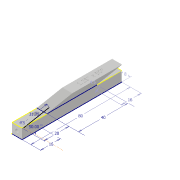
# Autodesk Inventor part: MineralStop1.25x50
Saved by Autodesk Inventor 2018 (Build 220112000, 112)
## iProperties
Created: 2018-12-12
Part Number: MineralStop1.25x50
Material: Generic
Document SubType Name: Modeling
Designer: ball
Density: 1 g/cm^3
Appearance: Default
Author: ball
Autodesk Inventor part; units mm, degrees
ref_plane "YZ Plane" through (0, 0, 0) normal (1, 0, 0) x (0, 1, 0)
ref_plane "XZ Plane" through (0, 0, 0) normal (0, 1, 0) x (-1, 0, 0)
ref_plane "XY Plane" through (0, 0, 0) normal (0, 0, 1) x (1, 0, 0)
sketch "Sketch1" plane through (0, 0, 0) normal (0, 1, 0) x (-1, 0, 0)
  line L0 (0, 0) -> (-8, 0)
  line L1 (-8, 0) -> (-8, -80)
  line L2 (-8, -80) -> (0, -80)
  line L3 (0, -80) -> (0, 0)
  circle A0 centre (-4, -16) radius 2.25
  circle A1 centre (-4, -64) radius 2.25
  circle A2 centre (-4, -16) radius 3.5 construction
  dimension "d0" = 8
  dimension "d1" = 80
  dimension "d6" = 4.5
  dimension "d7" = 4.5
  dimension "d26" = 16
  dimension "d27" = 16
  dimension "d43" = 7
  constraints: 8 end point, 3 centre point, 2 parallel, 1 coincident, 1 horizontal, 1 perpendicular
  measures "d0" distance of L2.end L1.end
  measures "d1" distance of L1.end L0.end
  measures "d6" diameter of A0
  measures "d7" diameter of A1
  measures "d26" distance from line of L0 A0.centre
  measures "d27" distance from line of L2 A1.centre
  measures "d43" diameter of A2
extrude "Extrusion1" [suppressed]
extrude "Extrusion2" add sketch "Sketch1" along normal blind 8
sketch "Sketch2" plane through (0, 0, 0) normal (0, 0, 1) x (1, 0, 0)
  circle A0 centre (4, 4) radius 1.35
  point P0 (0, 0)
  dimension "d10" = 2.7
  constraints: 1 centre point
  measures "d10" diameter of A0
hole "Hole1" at (4, 4, 0) direction (0, 0, -1) diameter 2.7 depth 10
sketch "Sketch3" plane through (8, 0, -80) normal (0, 0, -1) x (-1, 0, 0)
  circle A0 centre (4, 4) radius 1.35
  point P0 (8, 0)
  dimension "d18" = 2.7
  constraints: 1 centre point
  measures "d18" diameter of A0
hole "Hole2" at (4, 4, -80) direction (0, 0, 1) diameter 2.7 depth 10
sketch "Sketch5" plane through (0, 0, 0) normal (0, 0, 1) x (1, 0, 0)
  line L0 (9.3659, 8.9784) -> (29.7744, 33.3003)
  line L1 (9.3659, 8.9784) -> (41.1159, 8.9784) construction
  point P0 (0, 0)
  dimension "d33" = 31.75
  dimension "d34" = 50
  constraints: 4 end point, 1 equal length, 1 horizontal
  measures "d33" distance of L0.start L0.end
  measures "d34" angle of L1 L0
sketch "Sketch4" plane through (0, 8, 0) normal (0, 1, 0) x (1, 0, 0)
  line L0 (0, 80) -> (0, 0) projected
  line L1 (8, 0) -> (8, 80) projected
  line L2 (0, 60) -> (8, 60)
  line L3 (8, 60) -> (8, 20)
  line L4 (8, 20) -> (0, 20)
  line L5 (0, 20) -> (0, 60)
  line L6 (0, 0) -> (8, 0) projected
  line L7 (8, 80) -> (0, 80) projected
  dimension "d28" = 40
  dimension "d29" = 20
  constraints: 8 end point, 2 parallel, 2 point on line, 1 horizontal, 1 perpendicular
  measures "d28" distance of L2.end L3.end
  measures "d29" distance between parallel lines of L6 L4
sweep "Sweep1" add profiles "Sketch4" path "Sketch5" contours L2 L1 L4 L0
sweep "Sweep2" [suppressed]
sketch "Sketch6" plane through (20.4085, 32.3219, -60) normal (0, 1, 0) x (1, 0, 0)
  line L0 (2.4072, -31.6899) -> (2.4072, -9.1748) construction
  line L1 (2.4072, -9.1748) -> (5.6553, -9.1748) construction
  line L2 (5.6553, -9.1748) -> (5.6553, -31.6899) construction
  line L3 (5.6553, -31.6899) -> (2.4072, -31.6899) construction
  line L4 (5.591, -29.741) -> (5.591, -31.228)
  line L5 (5.591, -31.228) -> (5.2798, -31.228)
  line L6 (5.2798, -31.228) -> (5.2798, -30.6747)
  line L7 (5.2798, -30.6747) -> (3.2371, -30.6747)
  line L8 (3.2371, -30.6747) -> (3.2371, -31.228)
  line L9 (3.2371, -31.228) -> (2.958, -31.228)
  spline S0 degree 2 poles (2.958, -31.228) (2.958, -30.9143) (2.7802, -30.6179) (2.5332, -30.5981) knots 0 0 0 1 2 2 2
  line L10 (2.5332, -30.5981) -> (2.5332, -30.282)
  line L11 (2.5332, -30.282) -> (5.2798, -30.282)
  line L12 (5.2798, -30.282) -> (5.2798, -29.741)
  line L13 (5.2798, -29.741) -> (5.591, -29.741)
  line L14 (5.591, -28.5258) -> (5.591, -29.0149)
  line L15 (5.591, -29.0149) -> (5.0081, -29.0149)
  line L16 (5.0081, -29.0149) -> (5.0081, -28.5258)
  line L17 (5.0081, -28.5258) -> (5.591, -28.5258)
  line L18 (5.591, -26.0311) -> (5.591, -27.9108)
  line L19 (5.591, -27.9108) -> (5.1588, -27.9108)
  spline S1 degree 2 poles (5.1588, -27.9108) (4.9686, -27.7082) (4.6154, -27.3476) (4.4252, -27.1747) knots 0 0 0 1 2 2 2
  spline S2 degree 2 poles (4.4252, -27.1747) (4.0423, -26.8264) (3.5829, -26.572) (3.3384, -26.572) knots 0 0 0 1 2 2 2
  spline S3 degree 2 poles (3.3384, -26.572) (3.21, -26.572) (3.0173, -26.6511) (2.9555, -26.7227) knots 0 0 0 1 2 2 2
  spline S4 degree 2 poles (2.9555, -26.7227) (2.8938, -26.7943) (2.832, -26.982) (2.832, -27.0957) knots 0 0 0 1 2 2 2
  spline S5 degree 2 poles (2.832, -27.0957) (2.832, -27.2043) (2.8864, -27.4266) (2.9284, -27.5279) knots 0 0 0 1 2 2 2
  spline S6 degree 2 poles (2.9284, -27.5279) (2.963, -27.6144) (3.0618, -27.7749) (3.0963, -27.8243) knots 0 0 0 1 2 2 2
  line L20 (3.0963, -27.8243) -> (3.0963, -27.8465)
  line L21 (3.0963, -27.8465) -> (2.6616, -27.8465)
  spline S7 degree 2 poles (2.6616, -27.8465) (2.5999, -27.7206) (2.4788, -27.2686) (2.4788, -27.066) knots 0 0 0 1 2 2 2
  spline S8 degree 2 poles (2.4788, -27.066) (2.4788, -26.6387) (2.9308, -26.157) (3.3162, -26.157) knots 0 0 0 1 2 2 2
  spline S9 degree 2 poles (3.3162, -26.157) (3.4965, -26.157) (3.7978, -26.241) (3.9263, -26.3151) knots 0 0 0 1 2 2 2
  spline S10 degree 2 poles (3.9263, -26.3151) (4.0596, -26.3892) (4.3215, -26.6041) (4.4474, -26.7227) knots 0 0 0 1 2 2 2
  spline S11 degree 2 poles (4.4474, -26.7227) (4.6574, -26.9153) (5.1069, -27.3871) (5.2378, -27.5279) knots 0 0 0 1 2 2 2
  line L22 (5.2378, -27.5279) -> (5.2378, -26.0311)
  line L23 (5.2378, -26.0311) -> (5.591, -26.0311)
  spline S12 degree 2 poles (4.6228, -23.776) (4.8426, -23.776) (5.2181, -23.9167) (5.3564, -24.0452) knots 0 0 0 1 2 2 2
  spline S13 degree 2 poles (5.3564, -24.0452) (5.4947, -24.1736) (5.6553, -24.5565) (5.6553, -24.7936) knots 0 0 0 1 2 2 2
  spline S14 degree 2 poles (5.6553, -24.7936) (5.6553, -25.011) (5.5589, -25.4358) (5.4824, -25.5914) knots 0 0 0 1 2 2 2
  line L24 (5.4824, -25.5914) -> (5.0501, -25.5914)
  line L25 (5.0501, -25.5914) -> (5.0501, -25.5618)
  spline S15 degree 2 poles (5.0501, -25.5618) (5.0847, -25.5148) (5.1736, -25.3395) (5.2131, -25.2333) knots 0 0 0 1 2 2 2
  spline S16 degree 2 poles (5.2131, -25.2333) (5.2551, -25.1122) (5.3021, -24.9122) (5.3021, -24.7862) knots 0 0 0 1 2 2 2
  spline S17 degree 2 poles (5.3021, -24.7862) (5.3021, -24.6627) (5.2131, -24.4305) (5.1168, -24.3465) knots 0 0 0 1 2 2 2
  spline S18 degree 2 poles (5.1168, -24.3465) (5.0254, -24.27) (4.7834, -24.1909) (4.6203, -24.1909) knots 0 0 0 1 2 2 2
  spline S19 degree 2 poles (4.6203, -24.1909) (4.4573, -24.1909) (4.2498, -24.2798) (4.1807, -24.3638) knots 0 0 0 1 2 2 2
  spline S20 degree 2 poles (4.1807, -24.3638) (4.1041, -24.4503) (4.0399, -24.7071) (4.0399, -24.8628) knots 0 0 0 1 2 2 2
  spline S21 degree 2 poles (4.0399, -24.8628) (4.0399, -25.0307) (4.0917, -25.3642) (4.114, -25.4654) knots 0 0 0 1 2 2 2
  line L26 (4.114, -25.4654) -> (2.543, -25.4654)
  line L27 (2.543, -25.4654) -> (2.543, -23.7932)
  line L28 (2.543, -23.7932) -> (2.9012, -23.7932)
  line L29 (2.9012, -23.7932) -> (2.9012, -25.0727)
  line L30 (2.9012, -25.0727) -> (3.7138, -25.0727)
  spline S22 degree 2 poles (3.7138, -25.0727) (3.704, -24.9986) (3.6965, -24.8553) (3.6965, -24.7961) knots 0 0 0 1 2 2 2
  spline S23 degree 2 poles (3.6965, -24.7961) (3.6965, -24.5614) (3.7731, -24.2378) (3.8867, -24.0896) knots 0 0 0 1 2 2 2
  spline S24 degree 2 poles (3.8867, -24.0896) (4.0004, -23.939) (4.3462, -23.776) (4.6228, -23.776) knots 0 0 0 1 2 2 2
  line L31 (2.4072, -22.1087) -> (3.5928, -22.1976)
  line L32 (3.5928, -22.1976) -> (3.5928, -22.4668)
  line L33 (3.5928, -22.4668) -> (2.4072, -22.5558)
  line L34 (2.4072, -22.5558) -> (2.4072, -22.1087)
  line L35 (2.4072, -22.8793) -> (3.5928, -22.9683)
  line L36 (3.5928, -22.9683) -> (3.5928, -23.2375)
  line L37 (3.5928, -23.2375) -> (2.4072, -23.3264)
  line L38 (2.4072, -23.3264) -> (2.4072, -22.8793)
  line L39 (5.591, -18.5123) -> (5.591, -18.9841)
  line L40 (5.591, -18.9841) -> (4.7315, -19.5399)
  line L41 (4.7315, -19.5399) -> (5.591, -20.1104)
  line L42 (5.591, -20.1104) -> (5.591, -20.5476)
  line L43 (5.591, -20.5476) -> (4.4573, -19.7548)
  line L44 (4.4573, -19.7548) -> (3.3038, -20.5402)
  line L45 (3.3038, -20.5402) -> (3.3038, -20.0685)
  line L46 (3.3038, -20.0685) -> (4.156, -19.5152)
  line L47 (4.156, -19.5152) -> (3.3038, -18.9495)
  line L48 (3.3038, -18.9495) -> (3.3038, -18.5123)
  line L49 (3.3038, -18.5123) -> (4.4326, -19.3003)
  line L50 (4.4326, -19.3003) -> (5.591, -18.5123)
  spline S25 degree 2 poles (4.6228, -15.1136) (4.8426, -15.1136) (5.2181, -15.2544) (5.3564, -15.3828) knots 0 0 0 1 2 2 2
  spline S26 degree 2 poles (5.3564, -15.3828) (5.4947, -15.5113) (5.6553, -15.8941) (5.6553, -16.1313) knots 0 0 0 1 2 2 2
  spline S27 degree 2 poles (5.6553, -16.1313) (5.6553, -16.3486) (5.5589, -16.7735) (5.4824, -16.9291) knots 0 0 0 1 2 2 2
  line L51 (5.4824, -16.9291) -> (5.0501, -16.9291)
  line L52 (5.0501, -16.9291) -> (5.0501, -16.8994)
  spline S28 degree 2 poles (5.0501, -16.8994) (5.0847, -16.8525) (5.1736, -16.6771) (5.2131, -16.5709) knots 0 0 0 1 2 2 2
  spline S29 degree 2 poles (5.2131, -16.5709) (5.2551, -16.4499) (5.3021, -16.2498) (5.3021, -16.1238) knots 0 0 0 1 2 2 2
  spline S30 degree 2 poles (5.3021, -16.1238) (5.3021, -16.0003) (5.2131, -15.7682) (5.1168, -15.6842) knots 0 0 0 1 2 2 2
  spline S31 degree 2 poles (5.1168, -15.6842) (5.0254, -15.6076) (4.7834, -15.5286) (4.6203, -15.5286) knots 0 0 0 1 2 2 2
  spline S32 degree 2 poles (4.6203, -15.5286) (4.4573, -15.5286) (4.2498, -15.6175) (4.1807, -15.7015) knots 0 0 0 1 2 2 2
  spline S33 degree 2 poles (4.1807, -15.7015) (4.1041, -15.7879) (4.0399, -16.0448) (4.0399, -16.2004) knots 0 0 0 1 2 2 2
  spline S34 degree 2 poles (4.0399, -16.2004) (4.0399, -16.3684) (4.0917, -16.7018) (4.114, -16.8031) knots 0 0 0 1 2 2 2
  line L53 (4.114, -16.8031) -> (2.543, -16.8031)
  line L54 (2.543, -16.8031) -> (2.543, -15.1309)
  line L55 (2.543, -15.1309) -> (2.9012, -15.1309)
  line L56 (2.9012, -15.1309) -> (2.9012, -16.4104)
  line L57 (2.9012, -16.4104) -> (3.7138, -16.4104)
  spline S35 degree 2 poles (3.7138, -16.4104) (3.704, -16.3363) (3.6965, -16.193) (3.6965, -16.1337) knots 0 0 0 1 2 2 2
  spline S36 degree 2 poles (3.6965, -16.1337) (3.6965, -15.8991) (3.7731, -15.5755) (3.8867, -15.4273) knots 0 0 0 1 2 2 2
  spline S37 degree 2 poles (3.8867, -15.4273) (4.0004, -15.2766) (4.3462, -15.1136) (4.6228, -15.1136) knots 0 0 0 1 2 2 2
  spline S38 degree 2 poles (4.067, -12.777) (4.8871, -12.777) (5.6553, -13.2537) (5.6553, -13.7502) knots 0 0 0 1 2 2 2
  spline S39 degree 2 poles (5.6553, -13.7502) (5.6553, -14.254) (4.8723, -14.7258) (4.0695, -14.7258) knots 0 0 0 1 2 2 2
  spline S40 degree 2 poles (4.0695, -14.7258) (3.2445, -14.7258) (2.4813, -14.2491) (2.4813, -13.7502) knots 0 0 0 1 2 2 2
  spline S41 degree 2 poles (2.4813, -13.7502) (2.4813, -13.2487) (3.2717, -12.777) (4.067, -12.777) knots 0 0 0 1 2 2 2
  spline S42 degree 2 poles (4.9958, -13.3006) (4.8451, -13.2413) (4.3807, -13.1919) (4.067, -13.1919) knots 0 0 0 1 2 2 2
  spline S43 degree 2 poles (4.067, -13.1919) (3.7534, -13.1919) (3.2915, -13.2413) (3.1359, -13.3031) knots 0 0 0 1 2 2 2
  spline S44 degree 2 poles (3.1359, -13.3031) (2.9802, -13.3648) (2.8197, -13.5797) (2.8197, -13.7502) knots 0 0 0 1 2 2 2
  spline S45 degree 2 poles (2.8197, -13.7502) (2.8197, -13.9206) (2.9802, -14.1404) (3.1408, -14.2046) knots 0 0 0 1 2 2 2
  spline S46 degree 2 poles (3.1408, -14.2046) (3.2964, -14.2664) (3.7706, -14.3109) (4.0695, -14.3109) knots 0 0 0 1 2 2 2
  spline S47 degree 2 poles (4.0695, -14.3109) (4.3906, -14.3109) (4.8204, -14.2713) (4.9884, -14.2071) knots 0 0 0 1 2 2 2
  spline S48 degree 2 poles (4.9884, -14.2071) (5.1464, -14.1478) (5.3169, -13.928) (5.3169, -13.7502) knots 0 0 0 1 2 2 2
  spline S49 degree 2 poles (5.3169, -13.7502) (5.3169, -13.5822) (5.1563, -13.3624) (4.9958, -13.3006) knots 0 0 0 1 2 2 2
  spline S50 degree 2 poles (3.2692, -10.8429) (3.5977, -10.8429) (4.0473, -11.2925) (4.0473, -11.621) knots 0 0 0 1 2 2 2
  spline S51 degree 2 poles (4.0473, -11.621) (4.0473, -11.947) (3.6002, -12.4015) (3.2692, -12.4015) knots 0 0 0 1 2 2 2
  spline S52 degree 2 poles (3.2692, -12.4015) (2.9407, -12.4015) (2.4912, -11.952) (2.4912, -11.621) knots 0 0 0 1 2 2 2
  spline S53 degree 2 poles (2.4912, -11.621) (2.4912, -11.2925) (2.9407, -10.8429) (3.2692, -10.8429) knots 0 0 0 1 2 2 2
  spline S54 degree 2 poles (3.2692, -11.164) (3.0716, -11.164) (2.8024, -11.4259) (2.8024, -11.621) knots 0 0 0 1 2 2 2
  spline S55 degree 2 poles (2.8024, -11.621) (2.8024, -11.8186) (3.0716, -12.0804) (3.2692, -12.0804) knots 0 0 0 1 2 2 2
  spline S56 degree 2 poles (3.2692, -12.0804) (3.4693, -12.0804) (3.7361, -11.8137) (3.7361, -11.621) knots 0 0 0 1 2 2 2
  spline S57 degree 2 poles (3.7361, -11.621) (3.7361, -11.4259) (3.4644, -11.164) (3.2692, -11.164) knots 0 0 0 1 2 2 2
  point P0 (-20.4085, -60)
  constraints: 2 other
emboss "Emboss2" sketch "Sketch6" operation cut depth 1 direction (0, -1, 0)
body "Solid1"
